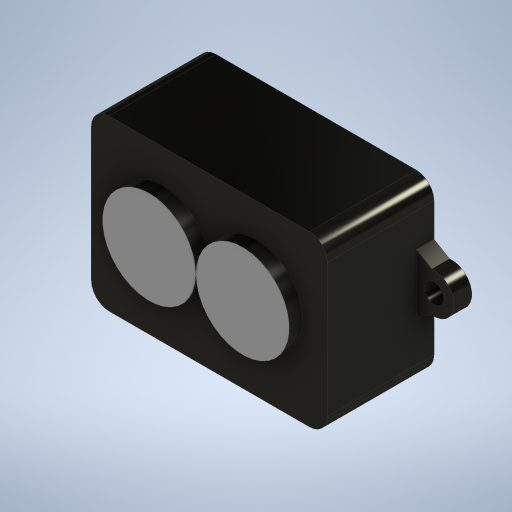
# Autodesk Inventor part: lidarsensor
Saved by Autodesk Inventor 2023.1 (Build 271208000, 208)
## iProperties
Created: 2023-03-22
Part Number: lidarsensor
Material: Generic
Document SubType Name: Modeling
Designer: liaar
Density: 1 g/cm^3
Appearance: Default
Author: liaar
Autodesk Inventor part; units mm, degrees
ref_plane "YZ Plane" through (0, 0, 0) normal (1, 0, 0) x (0, 1, 0)
ref_plane "XZ Plane" through (0, 0, 0) normal (0, 1, 0) x (-1, 0, 0)
ref_plane "XY Plane" through (0, 0, 0) normal (0, 0, 1) x (1, 0, 0)
sketch "Sketch1" plane through (0, 0, 0) normal (0, 0, 1) x (1, 0, 0)
  line L0 (2, 0) -> (24.5, 0)
  line L1 (26.5, 2) -> (26.5, 17)
  line L2 (24.5, 19) -> (2, 19)
  line L3 (0, 17) -> (0, 2)
  arc A0 (2, 19) -> (0, 17) centre (2, 17) ccw
  arc A1 (26.5, 17) -> (24.5, 19) centre (24.5, 17) ccw
  arc A2 (0, 2) -> (2, 0) centre (2, 2) ccw
  arc A3 (24.5, 0) -> (26.5, 2) centre (24.5, 2) ccw
  line L4 (4.25, 0) -> (22.25, 0)
  line L5 (22.25, 0) -> (22.25, -2.25)
  line L6 (22.25, -2.25) -> (4.25, -2.25)
  line L7 (4.25, -2.25) -> (4.25, 0)
  circle A4 centre (-2, 10) radius 1.1
  circle A5 centre (28.5, 10) radius 1.1
  arc A6 (-1.7552, 12.2366) -> (-1.7552, 7.7634) centre (-2, 10) ccw
  arc A7 (28.2552, 7.7634) -> (28.2552, 12.2366) centre (28.5, 10) ccw
  circle A8 centre (18.5, 10) radius 5.25
  circle A9 centre (8, 10) radius 5.25
  line L8 (-1.7552, 12.2366) -> (0, 13.25)
  line L9 (-1.7552, 7.7634) -> (0, 6.75)
  line L10 (13.25, 19) -> (13.25, 0) construction
  line L11 (28.2552, 12.2366) -> (26.5, 13.25)
  line L12 (28.2552, 7.7634) -> (26.5, 6.75)
  circle A10 centre (8, 10) radius 5
  circle A11 centre (18.5, 10) radius 5
  point P0 (0, 0)
  point P1 (26.5, 19)
  point P2 (26.5, 0)
  point P3 (0, 19)
  point P4 (13.25, 0)
  point P5 (13.25, -2.25)
  point P6 (13.25, 10)
  dimension "d10" = 10.5
  dimension "d11" = 10.5
  dimension "d0" = 26.5
  dimension "d1" = 19
  dimension "d2" = 2
  dimension "d3" = 21.25
  dimension "d4" = 18
  dimension "d5" = 2.2
  dimension "d6" = 4.5
  dimension "d7" = 4.5
  dimension "d8" = 9
  dimension "d9" = 30.5
  dimension "d12" = 10.5
  dimension "d13" = 15.25
  dimension "d14" = 60
  dimension "d15" = 60
  dimension "d16" = 3.25
  dimension "d17" = 3.25
  dimension "d18" = 10
  dimension "d19" = 10
  dimension "d20" = 60
  dimension "d21" = 60
  dimension "d22" = 3.25
  dimension "d23" = 3.25
  dimension "d24" = 10
  dimension "d25" = 10
  constraints: 26 end point, 13 point on line, 12 point on circle, 10 centre point, 8 tangent, 4 coincident, 4 equal radius, 4 midpoint, 4 parallel, 3 horizontal alignment, 2 horizontal, 2 perpendicular, 2 vertical alignment, 1 vertical, 4 other
  measures "d0" distance of point (26.5, 19) point (0, 19)
  measures "d1" distance of point (26.5, 0) point (26.5, 19)
  measures "d2" radius of A0
  measures "d3" distance between parallel lines of L2 L6
  measures "d4" distance between parallel lines of L5 L7
  measures "d5" diameter of A4
  measures "d6" diameter of A6
  measures "d7" diameter of A7
  measures "d8" distance from line of L2 A4.centre
  measures "d9" distance of A5.centre A4.centre
  measures "d12" distance of point (18.5, 10) point (8, 10)
  measures "d13" distance of point (13.25, 10) A4.centre
  measures "d14" angle of L8 L3
  measures "d15" angle of L3 L9
  measures "d16" vertical distance of L9.end A4.centre
  measures "d17" vertical distance of L8.end A4.centre
  measures "d18" distance from line of L0 point (8, 10)
  measures "d19" distance from line of L0 point (18.5, 10)
  measures "d20" angle of L11 L1
  measures "d21" angle of L1 L12
  measures "d22" vertical distance of L11.end A7.centre
  measures "d23" vertical distance of L12.end A5.centre
  measures "d24" diameter of A10
  measures "d25" diameter of A11
extrude "Extrusion1" add sketch "Sketch1" along normal blind 12 contours A2 L3 A0 L2 A1 L1 A3 L0
extrude "Extrusion2" add sketch "Sketch1" along normal blind 2 contours L9 A6 L8 L3 | L1 L11 A7 L12
extrude "Extrusion3" add sketch "Sketch1" along normal blind 8 contours L0 L5 L6 L7
fillet "Fillet1" radius 1 2 edges at (4.25, -1.125, 8) (22.25, -1.125, 8)
sketch "Sketch2" plane through (4.25, -2.25, 0) normal (0, -1, 0) x (1, 0, 0)
  line L0 (0, 0) -> (18, 0) projected
  line L1 (3.75, 0) -> (14.25, 0)
  line L2 (14.25, 0) -> (14.25, 5.8)
  line L3 (13.25, 6.8) -> (4.75, 6.8)
  line L4 (3.75, 5.8) -> (3.75, 0)
  line L5 (1, 8) -> (17, 8) projected
  arc A0 (4.75, 6.8) -> (3.75, 5.8) centre (4.75, 5.8) ccw
  arc A1 (14.25, 5.8) -> (13.25, 6.8) centre (13.25, 5.8) ccw
  point P0 (-4.25, 0)
  point P1 (9, 6.8)
  point P2 (9, 8)
  dimension "d33" = 6.8
  dimension "d35" = 10.5
  dimension "d36" = 1
  constraints: 8 end point, 4 point on circle, 4 tangent, 2 centre point, 2 midpoint, 2 parallel, 1 equal radius, 1 horizontal, 1 perpendicular, 1 point on line, 1 vertical alignment
  measures "d33" distance between parallel lines of L0 L3
  measures "d35" distance between parallel lines of L2 L4
  measures "d36" radius of A0
extrude "Extrusion4" cut sketch "Sketch2" against normal blind 1
extrude "Extrusion5" add sketch "Sketch1" along normal blind 13.5 contours A8 | A9 | A10 | A11
body "Solid1"
